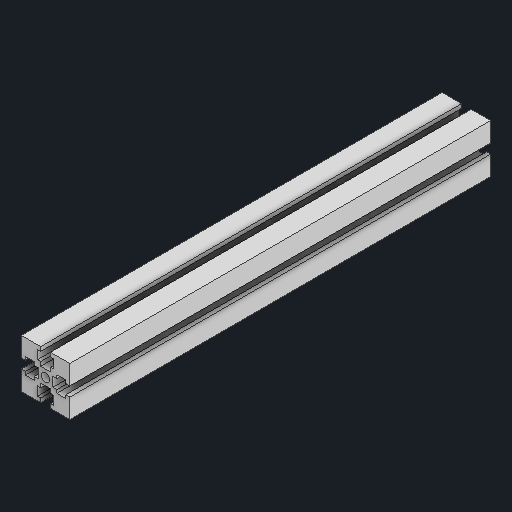
# Autodesk Inventor part: baicPart
Saved by Autodesk Inventor 2025.2 (Build 292293000, 293)
## iProperties
Company: FC-TORQUE
Created: 2025-03-14
Part Number: baicPart
Material: 一般
Document SubType Name: Modeling
Designer: Keito Tamura
Density: 1 g/cm^3
Appearance: 既定
Author: Keito Tamura
Autodesk Inventor part; units mm, degrees
ref_plane "YZ Plane" through (0, 0, 0) normal (1, 0, 0) x (0, 1, 0)
ref_plane "XZ Plane" through (0, 0, 0) normal (0, 1, 0) x (-1, 0, 0)
ref_plane "XY Plane" through (0, 0, 0) normal (0, 0, 1) x (1, 0, 0)
sketch "スケッチ1" plane through (0, 0, 0) normal (0, 0, 1) x (1, 0, 0)
  circle A0 centre (0, 0) radius 2.5
  line L0 (-15, 15) -> (15, 15)
  line L1 (15, 15) -> (15, -15)
  line L2 (15, -15) -> (-15, -15)
  line L3 (-15, -15) -> (-15, 15)
  line L4 (-15, 15) -> (15, -15) construction
  line L5 (15, 15) -> (-15, -15) construction
  line L6 (-3, 17.5) -> (3, 17.5)
  line L7 (3, 17.5) -> (3, 12.5)
  line L8 (3, 12.5) -> (-3, 12.5) construction
  line L9 (-3, 12.5) -> (-3, 17.5)
  line L10 (-3, 17.5) -> (3, 12.5) construction
  line L11 (3, 17.5) -> (-3, 12.5) construction
  line L12 (4.5, -4.5) -> (-4.5, -4.5)
  line L13 (-4.5, -4.5) -> (-4.5, 4.5)
  line L14 (-4.5, 4.5) -> (4.5, 4.5)
  line L15 (4.5, 4.5) -> (4.5, -4.5)
  line L16 (4.5, -4.5) -> (-4.5, 4.5) construction
  line L17 (-4.5, -4.5) -> (4.5, 4.5) construction
  line L18 (-7, 7) -> (7, 7)
  line L19 (7, 7) -> (7, -7)
  line L20 (7, -7) -> (-7, -7)
  line L21 (-7, -7) -> (-7, 7)
  line L22 (-7, 7) -> (7, -7) construction
  line L23 (7, 7) -> (-7, -7) construction
  line L24 (-7, 7) -> (-3, 7)
  line L25 (-3, 7) -> (-3, 3)
  line L26 (-3, 3) -> (-7, 3)
  line L27 (-7, 3) -> (-7, 7)
  line L28 (-7, -3) -> (-3, -3)
  line L29 (-3, -3) -> (-3, -7)
  line L30 (3, -7) -> (3, -3)
  line L31 (3, -3) -> (7, -3)
  line L32 (7, 3) -> (3, 3)
  line L33 (3, 3) -> (3, 7)
  line L34 (-15, 15) -> (-5, 15)
  line L35 (-5, 15) -> (-5, 5)
  line L36 (-5, 5) -> (-15, 5)
  line L37 (-15, 5) -> (-15, 15)
  line L38 (-15, -5) -> (-5, -5)
  line L39 (-5, -5) -> (-5, -15)
  line L40 (5, -15) -> (5, -5)
  line L41 (5, -5) -> (15, -5)
  line L42 (15, 5) -> (5, 5)
  line L43 (5, 5) -> (5, 15)
  line L44 (-3, 12.5) -> (-5, 12.5)
  line L45 (3, 12.5) -> (5, 12.5)
  line L46 (-12.5, -3) -> (-12.5, -5)
  line L47 (-12.5, -3) -> (-17.5, -3)
  line L48 (-17.5, 3) -> (-12.5, 3)
  line L49 (-12.5, 3) -> (-12.5, 5)
  line L50 (3, -12.5) -> (5, -12.5)
  line L51 (3, -12.5) -> (3, -17.5)
  line L52 (-3, -17.5) -> (-3, -12.5)
  line L53 (-3, -12.5) -> (-5, -12.5)
  line L54 (12.5, 3) -> (12.5, 5)
  line L55 (12.5, 3) -> (17.5, 3)
  line L56 (17.5, -3) -> (12.5, -3)
  line L57 (12.5, -3) -> (12.5, -5)
  point P0 (0, 15)
  point P1 (-7, 5)
  point P2 (-4.5, 3)
  point P3 (-4.5, -3)
  point P4 (-7, -5)
  point P5 (-15, -3)
  point P6 (-3, -15)
  point P7 (-5, -7)
  point P8 (-3, -4.5)
  point P9 (3, -4.5)
  point P10 (5, -7)
  point P11 (3, -15)
  point P12 (15, -3)
  point P13 (7, -5)
  point P14 (4.5, -3)
  point P15 (4.5, 3)
  point P16 (7, 5)
  point P17 (15, 3)
  point P18 (3, 15)
  point P19 (5, 7)
  point P20 (3, 4.5)
  point P21 (-3, 4.5)
  point P22 (-5, 7)
  point P23 (-3, 15)
  point P24 (-15, 3)
  dimension "d0" = 5
  dimension "d1" = 30
  dimension "d2" = 30
  dimension "d3" = 6
  dimension "d4" = 5
  dimension "d5" = 9
  dimension "d6" = 9
  dimension "d7" = 14
  dimension "d8" = 14
  dimension "d9" = 4
  dimension "d10" = 4
  dimension "d13" = 360
  dimension "d15" = 10
  dimension "d16" = 10
  dimension "d19" = 360
  dimension "d23" = 360
  constraints: 116 end point, 12 parallel, 9 midpoint, 8 perpendicular, 5 horizontal, 3 point on line, 1 centre point, 1 coincident, 83 other
  measures "d0" diameter of A0
  measures "d1" distance of L1.end L2.end
  measures "d2" distance of L0.end L1.end
  measures "d3" distance of L7.end L8.end
  measures "d4" distance of L6.end L7.end
  measures "d5" distance of L13.end L14.end
  measures "d6" distance of L12.end L13.end
  measures "d7" distance of L19.end L20.end
  measures "d8" distance of L18.end L19.end
  measures "d9" distance of L24.end L25.end
  measures "d10" distance between parallel lines of L25 L21
  measures "d15" distance of L35.end L36.end
  measures "d16" distance of L34.end L35.end
extrude "押し出し1" add sketch "スケッチ1" along normal blind 260 contours L0 L35 L18 L21 L36 L3 | L0 L9 L44 L35 | L36 L49 L48 L3 | L0 L43 L45 L7 | L35 L36 L21 L18 | L18 L25 L14 L13 L26 L21 L36 L35 | L47 L46 L38 L3 | L0 L1 L42 L19 L18 L43 | L38 L21 L20 L39 L2 L3 | L18 L43 L42 L19 L32 L15 L14 L33 | L25 L26 L13 L14 | L14 L33 L32 L15 L31 L30 L12 L29 L28 L13 L26 L25 | L28 L13 L12 L29 L20 L39 L38 L21 | L1 L55 L54 L42 | L18 L19 L42 L43 | L14 L15 L32 L33 | L39 L53 L52 L2 | L38 L39 L20 L21 | L28 L29 L12 L13 | L1 L41 L57 L56 | L51 L50 L40 L2 | L1 L2 L40 L20 L19 L41 | L31 L19 L41 L40 L20 L30 L12 L15 | L15 L12 L30 L31 | L19 L20 L40 L41
